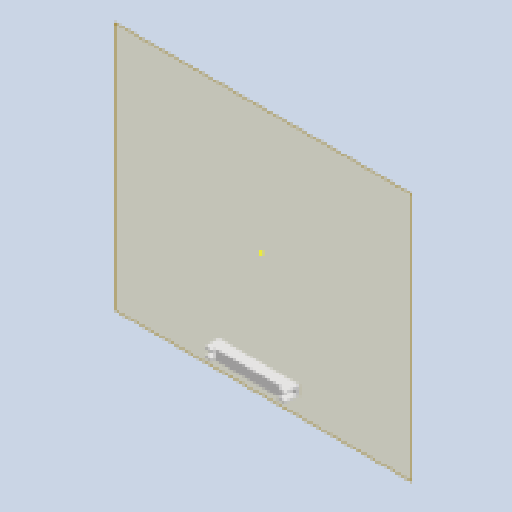
# Autodesk Inventor part: деталь держит провода
Saved by Autodesk Inventor 2024.2 (Build 282272000, 272)
## iProperties
Created: 2025-12-10
Part Number: деталь держит провода
Material: Типовые
Document SubType Name: Modeling
Designer: katya_notebook
Density: 1 g/cm^3
Appearance: По умолчанию
Author: katya_notebook
Autodesk Inventor part; units mm, degrees
ref_plane "YZ Plane" through (0, 0, 0) normal (1, 0, 0) x (0, 1, 0)
ref_plane "XZ Plane" through (0, 0, 0) normal (0, 1, 0) x (-1, 0, 0)
ref_plane "XY Plane" through (0, 0, 0) normal (0, 0, 1) x (1, 0, 0)
ref_plane "РабПлоскость1" through (0, 0, 0) normal (0, 0, 1) x (1, 0, 0)
sketch "Эскиз1" plane through (0, 0, 0) normal (0, 0, 1) x (1, 0, 0)
  line L0 (36.1495, -96.5) -> (-43.8505, -96.5)
  line L1 (-43.8505, -96.5) -> (-43.8505, -106.5)
  line L2 (-43.8505, -106.5) -> (36.1495, -106.5)
  line L3 (36.1495, -106.5) -> (36.1495, -96.5)
  line L4 (22.5, -91.5) -> (-22.5, -91.5) projected
  circle A0 centre (0, -101.5) radius 2
  circle A1 centre (22.5, -101.5) radius 2
  circle A2 centre (-22.5, -101.5) radius 2
  point P0 (0, 0)
  dimension "d0" = 80
  dimension "d1" = 10
  dimension "d2" = 5
  dimension "d3" = 4
  dimension "d5" = 4
  dimension "d6" = 4
  constraints: 8 end point, 3 centre point, 2 parallel, 1 horizontal, 1 perpendicular
  measures "d0" distance of L0.start L0.end
  measures "d1" distance of L2.end L0.start
  measures "d2" distance between parallel lines of L0 L4
  measures "d3" diameter of A0
  measures "d5" diameter of A1
  measures "d6" diameter of A2
extrude "Выдавливание1" add sketch "Эскиз1" along normal blind 2
sketch "Эскиз2" plane through (0, 0, 2) normal (0, 0, 1) x (1, 0, 0)
  point P0 (0, 0)
sketch "Эскиз3" plane through (-43.8505, -106.5, 0) normal (0, -1, 0) x (1, 0, 0)
  line L0 (0, 0) -> (0, 2) projected
  line L1 (0, 2) -> (0, 13.9799)
  line L2 (0, 13.9799) -> (7, 13.9799)
  line L3 (7, 13.9799) -> (7, 9)
  line L4 (7, 9) -> (73, 9)
  line L5 (73, 9) -> (73, 13.9799)
  line L6 (73, 13.9799) -> (80, 13.9799)
  line L7 (80, 13.9799) -> (80, 2)
  line L8 (0, 2) -> (80, 2)
  point P0 (43.8505, 0)
  point P1 (80, 2)
  dimension "d9" = 7
  dimension "d10" = 7
  dimension "d15" = 7
  constraints: 16 end point, 5 perpendicular, 2 point on line, 1 coincident, 1 horizontal, 1 vertical
  measures "d9" distance of L1.end L2.end
  measures "d10" distance of L5.end L6.end
  measures "d15" distance between parallel lines of L8 L4
extrude "Выдавливание2" add sketch "Эскиз3" against normal blind 2
sketch "Эскиз4" plane through (-43.8505, -96.5, 0) normal (0, 1, 0) x (1, 0, 0)
  line L0 (0, -2) -> (80, -2) projected
  line L1 (0, -2) -> (0, -13.9799) projected
  line L2 (0, -13.9799) -> (7, -13.9799) projected
  line L3 (7, -13.9799) -> (7, -9) projected
  line L4 (7, -9) -> (73, -9) projected
  line L5 (73, -9) -> (73, -13.9799) projected
  line L6 (73, -13.9799) -> (80, -13.9799) projected
  line L7 (80, -13.9799) -> (80, -2) projected
  point P0 (43.8505, 0)
extrude "Выдавливание3" add sketch "Эскиз4" against normal blind 2
sketch "Эскиз5" plane through (-36.8505, -96.5, 9) normal (0, 0, 1) x (1, 0, 0)
  line L0 (66, -10) -> (0, -10) projected
  line L1 (3.8262, -0.07) -> (63.012, -0.07)
  line L2 (63.012, -10) -> (3.8262, -10)
  line L3 (66, 0) -> (66, -2) projected
  line L4 (0, -10) -> (66, -10)
  line L5 (66, -10) -> (66, 0)
  line L6 (66, 0) -> (0, 0)
  line L7 (0, 0) -> (0, -10)
  point P0 (36.8505, 96.5)
  constraints: 12 end point, 3 parallel, 2 horizontal, 1 perpendicular, 1 point on line
extrude "Выдавливание4" add sketch "Эскиз5" along normal blind 2
